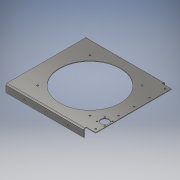
# Autodesk Inventor part: Turret Base Plate
Saved by Autodesk Inventor 2019.4 (Build 234330000, 330)
## iProperties
Created: 2020-01-11
Part Number: Turret Base Plate
Material: Steel, Mild
Document SubType Name: Sheet Metal
Designer: admin
Density: 7.85 g/cm^3
Sheet Metal Rule: Default_mm
Appearance: Semi-Polished
Mass: 823.421 g
Surface Area: 1091.07 cm^2
Volume: 104.894 cm^3
Author: admin
Autodesk Inventor part; units mm, degrees
ref_plane "YZ Plane" through (0, 0, 0) normal (1, 0, 0) x (0, 1, 0)
ref_plane "XZ Plane" through (0, 0, 0) normal (0, 1, 0) x (-1, 0, 0)
ref_plane "XY Plane" through (0, 0, 0) normal (0, 0, 1) x (1, 0, 0)
sketch "Sketch1" plane through (0, 0, 0) normal (0, 1, 0) x (-1, 0, 0)
  circle A0 centre (0, 0) radius 97.5
  line L0 (-140, 130) -> (140, 130)
  line L1 (140, 130) -> (140, -130)
  line L2 (140, -130) -> (-140, -130)
  line L3 (-140, -130) -> (-140, 130)
  line L4 (-140, 130) -> (140, -130) construction
  line L5 (140, 130) -> (-140, -130) construction
  dimension "d0" = 195
  dimension "d1" = 280
  dimension "d2" = 260
  measures "d0" diameter of A0
  measures "d1" distance of L1.end L2.end
  measures "d2" distance of L0.end L1.end
extrude "Plate1" add sketch "Sketch1" along normal blind 2
sketch "Sketch2" plane through (-140, 2, 128) normal (0, 0, 1) x (1, 0, 0)
  line L0 (280, 0) -> (0, 0)
  line L1 (0, 0) -> (0, -25)
  line L2 (0, -25) -> (280, -25)
  line L3 (280, -25) -> (280, 0)
  constraints: 6 end point, 1 horizontal, 1 perpendicular, 1 vertical
edge flange "Flange1" height 25 angle 90 thickness 2 bend radius 2 thickness toward (0, 0, 1) relief straight relief width 2 relief depth 1 corner gap 2 corner form 0 edges at (0, 0, 130) (0, 0, -130) wall of the first edge with corners at (140, 2, 128) (-140, 2, 128) (-140, -23, 128) (140, -23, 128)
bend "Bend1"
corner "Corner1"
unfold all bends "Unfold1" k factor 0.44 fixed face at (-125.8333, 2, 0)
sketch "Sketch3" plane through (0, 2, 0) normal (0, 1, 0) x (1, 0, 0)
  line L0 (140, -151.5239) -> (-140, -151.5239) projected
  line L1 (110, -151.5239) -> (110, -121.5239)
  line L2 (110, -121.5239) -> (140, -121.5239)
  line L3 (140, 126) -> (140, -126) projected
  line L4 (140, -126) -> (140, -130.5239) projected
  line L5 (140, -130.5239) -> (140, -151.5239) projected
  line L6 (-140, 151.5239) -> (140, 151.5239) projected
  line L7 (140, 151.5239) -> (110, 151.5239)
  line L8 (110, 151.5239) -> (110, 121.5239)
  line L9 (110, 121.5239) -> (140, 121.5239)
  line L10 (140, 121.5239) -> (140, 151.5239)
  point P0 (0, 0)
  dimension "d14" = 30
  dimension "d15" = 30
  dimension "d16" = 30
  dimension "d17" = 30
  constraints: 12 end point, 2 parallel, 2 perpendicular, 2 point on line, 1 horizontal, 1 vertical
  measures "d14" distance of L1.end L2.end
  measures "d15" distance of L1.start L1.end
  measures "d16" distance of L9.end L8.end
  measures "d17" distance of L8.end L7.end
extrude "Extrusion1" cut sketch "Sketch3" against normal through all
refold all bends "Refold1"
sketch "Sketch4" plane through (0, 2, 0) normal (0, 1, 0) x (1, 0, 0)
  circle A0 centre (0, 0) radius 133.75 construction
  circle A1 centre (123.7827, -76.187) radius 11.6 construction
  circle A2 centre (123.7827, -76.187) radius 12.75
  line L0 (123.7827, -76.187) -> (0, 0)
  line L1 (0, 0) -> (-154.4303, 0) construction
  line L2 (110, -130) -> (-140, -130) projected
  dimension "d20" = 25.5
  dimension "d21" = 267.5
  dimension "d22" = 23.2
  dimension "d27" = 53.813
  constraints: 4 end point, 3 centre point, 2 coincident, 1 horizontal, 1 tangent
  measures "d20" diameter of A2
  measures "d21" diameter of A0
  measures "d22" diameter of A1
  measures "d27" distance from line of L2 L0.start
extrude "Extrusion2" cut sketch "Sketch4" against normal through all
sketch "Sketch5" plane through (0, 2, 0) normal (0, 1, 0) x (1, 0, 0)
  circle A0 centre (123.7827, -76.187) radius 12.75 projected
  circle A1 centre (123.7827, -76.187) radius 17.5 construction
  circle A2 centre (136.1571, -63.8126) radius 2.25
  line L0 (111.4084, -88.5614) -> (136.1571, -88.5614) construction
  line L1 (136.1571, -88.5614) -> (136.1571, -63.8126) construction
  line L2 (136.1571, -63.8126) -> (111.4084, -63.8126) construction
  line L3 (111.4084, -63.8126) -> (111.4084, -88.5614) construction
  line L4 (111.4084, -88.5614) -> (136.1571, -63.8126) construction
  line L5 (136.1571, -88.5614) -> (111.4084, -63.8126) construction
  circle A3 centre (136.1571, -88.5614) radius 2.25
  circle A4 centre (111.4084, -88.5614) radius 2.25
  circle A5 centre (111.4084, -63.8126) radius 2.25
  point P0 (0, 0)
  dimension "d28" = 35
  dimension "d29" = 4.5
  dimension "d31" = 4.5
  dimension "d32" = 4.5
  dimension "d33" = 4.5
  constraints: 12 end point, 4 centre point, 4 coincident, 2 midpoint, 2 parallel, 2 perpendicular, 1 horizontal, 3 other
  measures "d29" diameter of A2
  measures "d31" diameter of A3
  measures "d32" diameter of A4
  measures "d33" diameter of A5
extrude "Extrusion3" cut sketch "Sketch5" against normal through all contours A2 | A3 | A4 | A5
sketch "Sketch6" plane through (0, 2, 0) normal (0, 1, 0) x (1, 0, 0)
  circle A0 centre (130, -111.5239) radius 2.75
  circle A1 centre (130, -38.4761) radius 2.75
  circle A2 centre (130, 11.5239) radius 2.75
  circle A3 centre (130, 111.5239) radius 2.75
  circle A4 centre (130, 61.5239) radius 2.75
  line L0 (130, -111.5239) -> (130, 111.5239) construction
  line L1 (110, -121.5239) -> (140, -121.5239) projected
  line L2 (140, 121.5239) -> (110, 121.5239) projected
  line L3 (140, 121.5239) -> (140, -121.5239) projected
  circle A5 centre (-128.612, 91) radius 2.75 projected
  circle A6 centre (-126.5993, -91) radius 2.75 projected
  point P0 (0, 0)
  dimension "d36" = 5.5
  dimension "d37" = 5.5
  dimension "d38" = 5.5
  dimension "d39" = 5.5
  dimension "d40" = 5.5
  dimension "d41" = 10
  dimension "d42" = 10
  dimension "d43" = 50
  dimension "d44" = 50
  dimension "d45" = 50
  dimension "d46" = 10
  constraints: 5 centre point, 3 point on line, 2 end point, 1 vertical
  measures "d36" diameter of A0
  measures "d37" diameter of A1
  measures "d38" diameter of A2
  measures "d39" diameter of A3
  measures "d40" diameter of A4
  measures "d41" distance from line of L1 L0.start
  measures "d42" distance from line of L2 L0.end
  measures "d43" distance of L0.end A4.centre
  measures "d44" distance of A4.centre A2.centre
  measures "d45" distance of A2.centre A1.centre
  measures "d46" distance between parallel lines of L3 L0
extrude "Extrusion4" cut sketch "Sketch6" against normal through all contours A0 | A1 | A2 | A3 | A4
sketch "Sketch7" plane through (-140, -23, 130) normal (0, 0, 1) x (1, 0, 0)
  circle A0 centre (60, 10) radius 2.75
  circle A1 centre (130, 10) radius 2.75
  circle A2 centre (200, 10) radius 2.75
  line L0 (250, 0) -> (0, 0) projected
  point P0 (140, 23)
  dimension "d49" = 5.5
  dimension "d50" = 5.5
  dimension "d51" = 5.5
  dimension "d52" = 10
  dimension "d53" = 10
  dimension "d54" = 10
  dimension "d56" = 70
  dimension "d57" = 70
  dimension "d58" = 50
  constraints: 3 centre point
  measures "d49" diameter of A0
  measures "d50" diameter of A1
  measures "d51" diameter of A2
  measures "d52" distance from line of L0 A0.centre
  measures "d53" distance from line of L0 A1.centre
  measures "d54" distance from line of L0 A2.centre
  measures "d56" distance of A1.centre A2.centre
  measures "d57" distance of A1.centre A0.centre
  measures "d58" horizontal distance of L0.start A2.centre
extrude "Extrusion5" cut sketch "Sketch7" against normal through all
sketch "Sketch8" plane through (0, 2, 0) normal (0, 1, 0) x (1, 0, 0)
  line L0 (-84, -84) -> (84, -84) construction
  line L1 (84, -84) -> (84, 84) construction
  line L2 (84, 84) -> (-84, 84) construction
  line L3 (-84, 84) -> (-84, -84) construction
  line L4 (-84, -84) -> (84, 84) construction
  line L5 (84, -84) -> (-84, 84) construction
  circle A0 centre (84, 84) radius 2.75
  circle A1 centre (-84, 84) radius 2.75
  circle A2 centre (-84, -84) radius 2.75
  circle A3 centre (84, -84) radius 2.75
  point P0 (0, 0)
  dimension "d61" = 168
  dimension "d62" = 168
  dimension "d63" = 5.5
  dimension "d64" = 5.5
  dimension "d65" = 5.5
  dimension "d66" = 5.5
  constraints: 12 end point, 4 centre point, 4 coincident, 2 midpoint, 2 parallel, 1 horizontal, 1 perpendicular
  measures "d61" distance of L2.end L1.end
  measures "d62" distance of L1.end L0.end
  measures "d63" diameter of A0
  measures "d64" diameter of A1
  measures "d65" diameter of A2
  measures "d66" diameter of A3
extrude "Extrusion6" cut sketch "Sketch8" against normal through all
equation "\"d3\" = Thickness"
equation "\"d4\" = BendReliefWidth"
equation "\"d5\" = BendReliefDepth"
equation "\"d6\" = MinimumRemnant"
equation "\"d7\" = TransitionRadius"
equation "\"d10\" = BendRadius"
equation "\"d11\" = CornerReliefSize"
equation "\"d12\" = GapSize"
equation "\"d13\" = JacobiRadiusSize"
equation "\"BendRadius\" = Thickness"
equation "\"BendReliefWidth\" = Thickness"
equation "\"BendReliefDepth\" = 0.5 * Thickness"
equation "\"CornerReliefSize\" = 4 * Thickness"
equation "\"MinimumRemnant\" = 2 * Thickness"
equation "\"TransitionRadius\" = BendRadius"
equation "\"JacobiRadiusSize\" = BendRadius"
equation "\"GapSize\" = Thickness"
equation "\"Thickness\" = 2"
body "Solid1"
